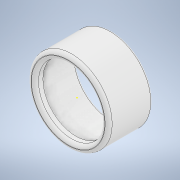
# Autodesk Inventor part: 5200_Biax_TxRx_Relative_Position_AirFlowGuide_MPSv2_v3
Saved by Autodesk Inventor 2021 (Build 250183000, 183)
## iProperties
Created: 2020-11-11
Part Number: 5200_Biax_TxRx_Relative_Position_AirFlowGuide_MPSv2_v3
Material: Acetal Resin, White
Document SubType Name: Modeling
Designer: Admin
Density: 1.425 g/cm^3
Appearance: Smooth - White
Author: Admin
Autodesk Inventor part; units mm, degrees
ref_plane "YZ Plane" through (0, 0, 0) normal (1, 0, 0) x (0, 1, 0)
ref_plane "XZ Plane" through (0, 0, 0) normal (0, 1, 0) x (-1, 0, 0)
ref_plane "XY Plane" through (0, 0, 0) normal (0, 0, 1) x (1, 0, 0)
sketch "Sketch1" plane through (0, 0, 0) normal (0, 0, 1) x (1, 0, 0)
  point P0 (0, 0)
sketch "Sketch2" plane through (0, 0, 0) normal (0, 0, 1) x (1, 0, 0)
  circle A0 centre (0, 0) radius 18.8587
  circle A1 centre (0, 0) radius 20.6375
  dimension "d0" = 37.7174
  dimension "d1" = 41.275
  constraints: 2 centre point, 2 coincident
  measures "d0" diameter of A0
  measures "d1" diameter of A1
extrude "Extrusion1" add sketch "Sketch2" along normal blind 5
sketch "Sketch3" plane through (0, 0, 0) normal (0, 0, -1) x (-1, 0, 0)
  circle A0 centre (0, 0) radius 20.6375
  circle A1 centre (0, 0) radius 23.1375
  dimension "d4" = 46.275
  constraints: 2 centre point, 2 coincident
  measures "d4" diameter of A1
extrude "Extrusion2" add sketch "Sketch3" along normal blind 20 and the other way blind 5
fillet "Fillet5" radius 1 2 edges at (20.6375, 0, -20) (23.1375, 0, -20)
fillet "Fillet6" radius 2 2 edges at (-18.8587, 0, 5) (23.1375, 0, 5)
fillet "Fillet7" radius 0.5 1 edges at (-18.8587, 0, 0)
body "Solid1"
